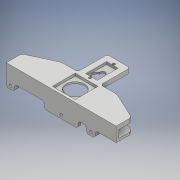
# Autodesk Inventor part: RescueKitThrow_slope
Saved by Autodesk Inventor 2018.3 (Build 223284000, 284)
## iProperties
Created: 2019-02-15
Part Number: RescueKitThrow_slope
Material: 一般
Document SubType Name: Modeling
Designer: TOMOKI
Density: 1 g/cm^3
Appearance: 既定
Author: TOMOKI
Autodesk Inventor part; units mm, degrees
ref_plane "YZ Plane" through (0, 0, 0) normal (1, 0, 0) x (0, 1, 0)
ref_plane "XZ Plane" through (0, 0, 0) normal (0, 1, 0) x (-1, 0, 0)
ref_plane "XY Plane" through (0, 0, 0) normal (0, 0, 1) x (1, 0, 0)
sketch "スケッチ7" plane through (0, 0, 0) normal (0, 0, 1) x (1, 0, 0)
  line L0 (0, 0) -> (130, 0)
  line L1 (130, 0) -> (130, 12)
  line L2 (0, 12) -> (0, 0)
  arc A0 (36.4343, 12) -> (93.5657, 12) centre (65, 40) ccw
  line L3 (130, 12) -> (93.5657, 12)
  line L4 (36.4343, 12) -> (0, 12)
  point P0 (65, 0)
  dimension "d17" = 130
  dimension "d18" = 12
  constraints: 10 end point, 3 perpendicular, 3 point on circle, 1 centre point, 1 horizontal, 1 midpoint, 1 parallel
  measures "d17" distance of L2.start L1.end
  measures "d18" distance of L1.end L0.end
extrude "押し出し6" add sketch "スケッチ7" against normal blind 14
sketch "スケッチ9" plane through (0, 0, 0) normal (0, 0, 1) x (1, 0, 0)
  line L0 (130, 0) -> (0, 0) projected
  line L1 (130, 0) -> (0, 0)
  line L2 (0, 0) -> (0, 30)
  line L3 (130, 30) -> (130, 0)
  arc A0 (65, 0) -> (93.5657, 12) centre (65, 40) ccw
  arc A1 (36.4343, 12) -> (65, 0) centre (65, 40) ccw projected
  line L4 (0, 30) -> (36.4343, 30)
  line L5 (93.5657, 30) -> (130, 30)
  line L6 (78.5, 0) -> (51.5, 0)
  line L7 (51.5, 0) -> (51.5, 27)
  line L8 (51.5, 27) -> (78.5, 27)
  line L9 (78.5, 27) -> (78.5, 0)
  line L10 (36.4343, 30) -> (49.4343, 30)
  line L11 (93.5657, 30) -> (86.5657, 30)
  arc A2 (68.0605, 45.5067) -> (61.9395, 45.5067) centre (65, 46) ccw
  arc A3 (61.9395, 45.5067) -> (68.0605, 45.5067) centre (65, 40) ccw
  line L12 (78.5, 65) -> (51.5, 65)
  line L13 (86.5657, 30) -> (80.4919, 30)
  line L14 (49.4343, 30) -> (51.5, 30)
  line L15 (78.5, 30) -> (80.4919, 30)
  line L16 (51.5, 30) -> (51.5, 65)
  line L17 (51.5, 65) -> (78.5, 65)
  line L18 (78.5, 65) -> (78.5, 30)
  dimension "d35" = 30
  dimension "d62" = 27
  dimension "d119" = 25
  dimension "d120" = 19
  dimension "d121" = 13.5
  dimension "d122" = 13.5
  dimension "d123" = 6.3
  dimension "d124" = 35
  dimension "d125" = 27
  dimension "d126" = 35
  dimension "d127" = 38
  dimension "d128" = 3.1
  constraints: 36 end point, 8 parallel, 7 horizontal, 6 point on circle, 3 centre point, 3 point on line, 2 perpendicular, 1 coincident
  measures "d35" distance of L0.end L2.end
  measures "d62" distance of L6.end L7.end
  measures "d119" distance from line of L12 A0.centre
  measures "d120" distance from line of L12 A2.centre
  measures "d121" distance from line of L16 A2.centre
  measures "d122" distance from line of L16 A0.centre
  measures "d123" radius of A3
  measures "d124" distance of L14.end L12.end
  measures "d125" distance of L12.start L12.end
  measures "d126" distance of L12.start L15.start
  measures "d127" distance between parallel lines of L8 L12
  measures "d128" radius of A2
extrude "押し出し7" add sketch "スケッチ9" against normal blind 5 contours L0 L9 L8 L7 L2 L4 L10 L14 L16 L12 L18 L15 L13 L11 L5 L3
sketch "スケッチ11" plane through (0, 0, 0) normal (0, 0, 1) x (1, 0, 0)
  line L0 (0, 0) -> (130, 0) projected
  line L1 (0, 0) -> (130, 0)
  line L2 (130, 0) -> (130, -3)
  line L3 (130, -3) -> (0, -3)
  line L4 (0, -3) -> (0, 0)
  point P0 (65, 0)
  dimension "d29" = 130
  dimension "d30" = 3
  constraints: 8 end point, 2 parallel, 1 horizontal, 1 perpendicular
  measures "d29" distance of L2.end L3.end
  measures "d30" distance of L0.end L2.end
extrude "押し出し9" add sketch "スケッチ11" against normal blind 14
sketch "スケッチ12" plane through (0, 0, -14) normal (0, 0, -1) x (-1, 0, 0)
  line L0 (-130, 12) -> (-130, -3) projected
  line L1 (0, -3) -> (0, 12) projected
  line L2 (-93.5657, 12) -> (-130, 12) projected
  line L3 (0, 12) -> (-36.4343, 12) projected
  line L4 (-93.5657, 12) -> (-130, 0)
  line L5 (-130, 12) -> (-130, -3) projected
  line L6 (-36.4343, 12) -> (0, 0)
  line L7 (0, -3) -> (0, 12) projected
  line L8 (0, 12) -> (0, 0)
  line L9 (-130, 0) -> (-130, 12)
  line L10 (-130, 12) -> (-93.5657, 12)
  line L11 (-36.4343, 12) -> (0, 12)
  arc A0 (-93.5657, 12) -> (-36.4343, 12) centre (-65, 40) ccw projected
  line L12 (-130, -3) -> (0, -3) projected
  constraints: 12 end point, 2 horizontal, 2 perpendicular, 2 point on line, 1 parallel
extrude "押し出し10" cut sketch "スケッチ12" against normal blind 9 contours L2 L4 L0 | L3 L1 L6
sketch "スケッチ13" plane through (0, 0, 0) normal (0, 0, 1) x (1, 0, 0)
  arc A0 (70.25, 42.9047) -> (70.25, 37.0953) centre (65, 40) ccw projected
  line L0 (58.15, 57.442) -> (58.15, 32.742)
  line L1 (58.15, 32.742) -> (71.85, 32.742)
  line L2 (71.85, 32.742) -> (71.85, 57.442)
  line L3 (71.85, 57.442) -> (58.15, 57.442)
  point P0 (0, 0)
  point P1 (36.4343, 50)
  dimension "d47" = 24.7
  dimension "d48" = 13.7
  constraints: 8 end point, 2 parallel, 1 perpendicular
  measures "d47" distance of L2.end L1.end
  measures "d48" distance of L1.end L0.end
extrude "押し出し11" cut sketch "スケッチ13" against normal blind 3
sketch "スケッチ14" plane through (0, 0, 0) normal (0, 0, 1) x (1, 0, 0)
  arc A0 (68.0605, 45.5067) -> (61.9395, 45.5067) centre (65, 46) ccw projected
  circle A1 centre (65, 31) radius 1.5
  circle A2 centre (65, 59.2) radius 1.5
  point P0 (0, 0)
  dimension "d86" = 3
  constraints: 2 centre point
  measures "d86" diameter of A2
extrude "押し出し12" cut sketch "スケッチ14" against normal blind 10
sketch "スケッチ15" plane through (0, 0, 0) normal (0, 0, 1) x (1, 0, 0)
  arc A0 (51.5, 2.347) -> (78.5, 2.347) centre (65, 40) ccw projected
  line L0 (0, 30) -> (0, -3) projected
  line L1 (0, -3) -> (130, -3) projected
  line L2 (130, -3) -> (130, 30) projected
  line L3 (51.5, 27) -> (78.5, 27)
  line L4 (78.5, 27) -> (78.5, 0)
  line L5 (78.5, 0) -> (51.5, 0)
  line L6 (51.5, 0) -> (51.5, 27)
  line L7 (51.5, 2.347) -> (51.5, 27) projected
  line L8 (51.5, 27) -> (78.5, 27) projected
  line L9 (78.5, 27) -> (78.5, 2.347) projected
  line L10 (130, 30) -> (78.5, 30) projected
  line L11 (78.5, 30) -> (78.5, 65) projected
  line L12 (78.5, 65) -> (51.5, 65) projected
  line L13 (51.5, 65) -> (51.5, 30) projected
  line L14 (51.5, 30) -> (0, 30) projected
  point P0 (0, 0)
  dimension "d63" = 27
  dimension "d64" = 27
  constraints: 8 end point, 2 parallel, 1 horizontal, 1 perpendicular
  measures "d63" distance of L4.end L5.end
  measures "d64" distance of L3.end L4.end
extrude "押し出し13" cut sketch "スケッチ15" against normal blind 5 contours L6 L3 L4 A0 | A0 L5 L6 | A0 L4 L5
sketch "スケッチ16" plane through (0, 0, -5) normal (0, 0, -1) x (-1, 0, 0)
  line L0 (-78.5, 27) -> (-51.5, 27) projected
  line L1 (-78.5, 2.347) -> (-78.5, 27) projected
  line L2 (-51.5, 27) -> (-51.5, 2.347) projected
  line L3 (-65, 0) -> (-51.5, 0) projected
  line L4 (-78.5, 0) -> (-65, 0) projected
  circle A0 centre (-65, 13.5) radius 11
  line L5 (-78.5, 27) -> (-51.5, 27)
  line L6 (-51.5, 27) -> (-51.5, -1)
  line L7 (-51.5, -1) -> (-78.5, -1)
  line L8 (-78.5, -1) -> (-78.5, 27)
  point P0 (0, 0)
  dimension "d67" = 22
  dimension "d68" = 13.5
  dimension "d69" = 13.5
  dimension "d70" = 27
  dimension "d71" = 28
  constraints: 8 end point, 2 parallel, 1 centre point, 1 horizontal, 1 perpendicular
  measures "d67" diameter of A0
  measures "d68" distance from line of A0.centre L2
  measures "d69" distance from line of L0 A0.centre
  measures "d70" distance of L6.end L7.end
  measures "d71" distance of L5.end L6.end
extrude "押し出し14" add sketch "スケッチ16" against normal blind 2
sketch "スケッチ17" plane through (0, 0, -14) normal (0, 0, -1) x (-1, 0, 0)
  line L0 (0, -3) -> (-130, -3) projected
  line L1 (0, 30) -> (-51.5, 30) projected
  line L2 (-130, -3) -> (0, -3)
  line L3 (0, -3) -> (0, 30)
  line L4 (0, 30) -> (-130, 30)
  line L5 (-130, 30) -> (-130, -3)
  line L6 (0, 0) -> (-36.4343, 12) projected
  line L7 (-93.5657, 12) -> (-130, 0) projected
  line L8 (-36.4343, -3) -> (-93.5657, -3)
  line L9 (-93.5657, 30) -> (-36.4343, 30)
  arc A0 (-61.9395, 45.5067) -> (-68.0605, 45.5067) centre (-65, 46) ccw projected
  arc A1 (-93.5657, 25.584) -> (-36.4343, 25.584) centre (-65, 49.1) ccw
  line L10 (-130, 0) -> (-130, 30) projected
  line L11 (-130, 25.584) -> (-93.5657, 25.584)
  line L12 (-36.4343, 25.584) -> (0, 25.584)
  arc A2 (-93.5657, 12) -> (-36.4343, 12) centre (-65, 40) ccw projected
  line L13 (-130, 0) -> (-130, -3) projected
  line L14 (-130, -3) -> (0, -3) projected
  line L15 (0, -3) -> (0, 0) projected
  point P0 (-49.4343, 30)
  dimension "d118" = 74
  constraints: 16 end point, 4 point on line, 3 parallel, 3 perpendicular, 3 point on circle, 2 horizontal, 1 centre point
  measures "d118" diameter of A1
extrude "押し出し15" add sketch "スケッチ17" along normal blind 3 contours L0 L5 L7 A2 L6 L3 | L6 A2 L7 L5 L11 A1 L12 L3
sketch "スケッチ18" plane through (0, 0, -17) normal (0, 0, -1) x (-1, 0, 0)
  line L0 (-130, -3) -> (0, -3) projected
  line L1 (-10, -3) -> (0, -3)
  line L2 (0, -3) -> (0, 2)
  line L3 (0, 2) -> (-10, 2)
  line L4 (-10, 2) -> (-10, -3)
  line L5 (-95, -3) -> (-105, -3)
  line L6 (-105, -3) -> (-105, 2)
  line L7 (-105, 2) -> (-95, 2)
  line L8 (-95, 2) -> (-95, -3)
  line L9 (0, -3) -> (0, 25.584) projected
  line L10 (-130, 25.584) -> (-130, -3) projected
  line L11 (-130, 25.584) -> (-130, -3) projected
  line L12 (-130, -3) -> (0, -3) projected
  line L13 (0, -3) -> (0, 25.584) projected
  line L14 (-85, -3) -> (-45, -3)
  line L15 (-45, -3) -> (-45, 0)
  line L16 (-45, 0) -> (-85, 0)
  line L17 (-85, 0) -> (-85, -3)
  line L18 (0, 25.584) -> (-36.4343, 25.584) projected
  arc A0 (-93.5657, 25.584) -> (-36.4343, 25.584) centre (-65, 49.1) ccw projected
  line L19 (-93.5657, 25.584) -> (-130, 25.584) projected
  point P0 (0, 0)
  point P1 (0, 30)
  point P2 (-130, 30)
  dimension "d87" = 10
  dimension "d88" = 5
  dimension "d89" = 10
  dimension "d90" = 5
  dimension "d97" = 0
  dimension "d109" = 25
  dimension "d110" = 40
  constraints: 24 end point, 6 parallel, 3 horizontal, 3 perpendicular, 1 point on line
  measures "d87" distance of L3.end L2.end
  measures "d88" distance of L2.end L1.end
  measures "d89" distance of L6.end L7.end
  measures "d90" distance of L5.end L6.end
  measures "d97" distance between parallel lines of L2 L9
  measures "d109" distance between parallel lines of L10 L6
  measures "d110" distance of L16.end L15.end
extrude "押し出し16" add sketch "スケッチ18" along normal blind 8 contours L6 L7 L8 L0 | L17 L16 L15 L0 | L4 L3 L2 L0
sketch "スケッチ19" plane through (0, 2, -17) normal (0, 1, 0) x (1, 0, 0)
  line L0 (10, 0) -> (0, 0) projected
  line L1 (10, 0) -> (10, 8) projected
  line L2 (0, 8) -> (10, 8) projected
  line L3 (0, 0) -> (0, 8) projected
  line L4 (105, 0) -> (95, 0) projected
  line L5 (105, 0) -> (105, 8) projected
  line L6 (95, 8) -> (105, 8) projected
  line L7 (95, 0) -> (95, 8) projected
  circle A0 centre (5, 4) radius 1.6
  circle A1 centre (100, 4) radius 1.6
  line L8 (85, 0) -> (45, 0) projected
  line L9 (85, 0) -> (85, 8) projected
  line L10 (45, 8) -> (85, 8) projected
  line L11 (45, 0) -> (45, 8) projected
  circle A2 centre (65, 4) radius 1.6
  point P0 (0, -17)
  dimension "d93" = 3.2
  dimension "d99" = 3.2
  dimension "d100" = 5
  dimension "d111" = 3.2
  constraints: 3 centre point
  measures "d93" diameter of A0
  measures "d99" diameter of A1
  measures "d100" distance from line of L5 A1.centre
  measures "d111" diameter of A2
extrude "押し出し17" cut sketch "スケッチ19" against normal blind 8 contours A0 | A1 | A2
sketch "スケッチ20" plane through (0, 0, -17) normal (0, 0, -1) x (-1, 0, 0)
  line L0 (-130, 0) -> (-130, 30) projected
  line L1 (-130, 15) -> (-97.8324, 30)
  line L2 (-130, 30) -> (-78.5, 30) projected
  line L3 (-130, 15) -> (-94.507, 15) construction
  line L4 (0, 30) -> (0, -3) projected
  line L5 (0, 15) -> (-32.1676, 30)
  line L6 (-51.5, 30) -> (0, 30) projected
  line L7 (0, 15) -> (35.493, 15) construction
  point P0 (0, 0)
  point P1 (-80.4919, 30)
  point P2 (-49.4343, 30)
  point P3 (-130, 12)
  point P4 (0, 12)
  dimension "d101" = 25
  dimension "d102" = 155
  constraints: 8 end point, 3 point on line, 2 equal length, 2 horizontal, 1 midpoint
  measures "d101" angle of L3 L1
  measures "d102" angle of L7 L5
extrude "押し出し18" cut sketch "スケッチ20" against normal blind 20
chamfer "面取り1" distance 2 angle 45 14 edges at (95, -0.5, -25) (105, -0.5, -25) (10, -0.5, -25) (0, -0.5, -25) (5, 2, -17) (10, -0.5, -17) (100, 2, -17) (95, -0.5, -17) (105, -0.5, -17) (45, -1.5, -17) (65, 0, -17) (45, -1.5, -25) (85, -1.5, -25) (85, -1.5, -17)
chamfer "面取り2" distance 2 angle 45 8 edges at (51.5, 65, -2.5) (78.5, 65, -2.5) (0, 15, -2.5) (0, 15, -15.5) (130, 15, -2.5) (130, 15, -15.5) (78.5, 30, -2.5) (51.5, 30, -2.5)
chamfer "面取り3" distance 2 angle 45 6 edges at (32.1676, 30, -2.5) (97.8324, 30, -2.5) (107.3024, 25.584, -15.5) (22.6976, 25.584, -15.5) (36.4343, 25.584, -15.5) (93.5657, 25.584, -15.5)
equation "\"d25\" = d39"
equation "\"d39\" = 5"
